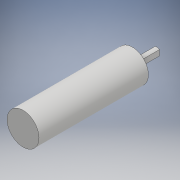
# Autodesk Inventor part: maxon_motor
Saved by Autodesk Inventor 2017 (Build 210142000, 142)
## iProperties
Part Number: maxon_motor
Material: 常规
Document SubType Name: Modeling
Designer: PS
Density: 1 g/cm^3
Appearance: 默认
Author: PS
Autodesk Inventor part; units mm, degrees
ref_plane "YZ Plane" through (0, 0, 0) normal (1, 0, 0) x (0, 1, 0)
ref_plane "XZ Plane" through (0, 0, 0) normal (0, 1, 0) x (-1, 0, 0)
ref_plane "XY Plane" through (0, 0, 0) normal (0, 0, 1) x (1, 0, 0)
sketch "草图1" plane through (0, 0, 0) normal (0, 1, 0) x (-1, 0, 0)
  circle A0 centre (0, 0) radius 6.5
  dimension "d0" = 13
  constraints: 1 centre point, 1 coincident
  measures "d0" diameter of A0
extrude "拉伸1" add sketch "草图1" along normal blind 44.5
sketch "草图2" plane through (0, 44.5, 0) normal (0, 1, 0) x (1, 0, 0)
  circle A0 centre (0, 0) radius 3
  dimension "d3" = 6
  constraints: 1 centre point, 1 coincident
  measures "d3" diameter of A0
extrude "拉伸2" add sketch "草图2" along normal blind 1
sketch "草图3" plane through (0, 45.5, 0) normal (0, 1, 0) x (1, 0, 0)
  circle A0 centre (0, 0) radius 2.5
  dimension "d6" = 5
  constraints: 1 centre point, 1 coincident
  measures "d6" diameter of A0
extrude "拉伸3" add sketch "草图3" along normal blind 1.5
sketch "草图4" plane through (0, 47, 0) normal (0, 1, 0) x (1, 0, 0)
  circle A0 centre (0, 0) radius 1.5
  dimension "d9" = 3
  constraints: 1 centre point, 1 coincident
  measures "d9" diameter of A0
extrude "拉伸4" add sketch "草图4" along normal blind 7.5
sketch "草图5" plane through (0, 54.5, 0) normal (0, 1, 0) x (1, 0, 0)
  circle A0 centre (0, 0) radius 1.5 projected
  line L0 (0, 0) -> (1, 0)
  line L1 (0, 0) -> (-1, 0)
  line L2 (-1, 0) -> (-1, 1.118)
  circle A1 centre (0, 0) radius 1.5 projected
  line L3 (-1, 0) -> (-1, -1.118)
  line L4 (1, 0) -> (1, -1.118)
  line L5 (1, 0) -> (1, 1.118)
  line L6 (-1, -1.118) -> (-1, 1.118)
  line L7 (1, 1.118) -> (1, -1.118)
  arc A2 (1, -1.118) -> (1, 1.118) centre (0, 0) ccw
  arc A3 (-1, 1.118) -> (-1, -1.118) centre (0, 0) ccw
  dimension "d12" = 1
  dimension "d13" = 1
  dimension "d14" = 1.5
  dimension "d15" = 1.5
  constraints: 16 end point, 12 point on circle, 4 perpendicular, 2 centre point, 2 horizontal, 1 parallel, 1 vertical
  measures "d12" distance of L0.start L0.end
  measures "d13" distance of L0.start L1.end
  measures "d14" radius of A2
  measures "d15" radius of A3
extrude "拉伸5" cut sketch "草图5" against normal up to surface (7.5 mm away) contours A0 L4 L5 | L2 L3 A0
sketch "草图6" plane through (0, 44.5, 0) normal (0, 1, 0) x (1, 0, 0)
  circle A0 centre (0, 0) radius 3 projected
  circle A1 centre (0, 0) radius 6.5 projected
  line L0 (0, 0) -> (-4.75, 0)
  line L1 (0, 0) -> (4.75, 0)
  circle A2 centre (-4.75, 0) radius 1
  circle A3 centre (4.75, 0) radius 1
  dimension "d18" = 4.75
  dimension "d19" = 4.75
  dimension "d20" = 2
  dimension "d21" = 2
  constraints: 4 end point, 2 centre point, 2 coincident, 2 horizontal
  measures "d18" distance of L0.start L0.end
  measures "d19" distance of L0.start L1.end
  measures "d20" diameter of A2
  measures "d21" diameter of A3
extrude "拉伸6" cut sketch "草图6" against normal blind 5 contours A2 | A3
